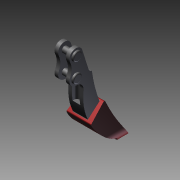
# Autodesk Inventor part: 205-S-HG
Saved by Autodesk Inventor 2011 SP1 (Build 150282100, 282)
## iProperties
Created: 2017-03-01
Part Number: 205-S-HG
Catalog Web Link: www.cadenas.de
Description: HG-SU-Handgriff
Vendor: DESTACO
Document SubType Name: Modeling
Designer: psAdmin
Manufacturer: DESTACO
Mass: 1.83339 g
Surface Area: 15.2284 cm^2
Volume: 1.83339 cm^3
Density: 1 g/cm^3
Category: PARTsolutions
Company: DESTACO
Title: 205-S-HG
Author: Cadenas PARTsolutions
Comments: Handgriff
PSOL_IDENT_0: {$CADENAS_DATA\23d-libs\destaco\destaco_gmbh\man_spann\horizontalspanner\standard\su_parts\handgriff
PSOL_IDENT_1: _su.prj},159 {VTYP=3D},{NB=205-S-HG},{LINA=205-S-HG},{NN=HG-SU},{DATE=20.09.2016 07:53:12},{GEOMDATE=
PSOL_IDENT_2: 01.12.2015 13:32:00},{VERSION=v1},{LINEID=20},{LINESUBID=-1},{WBVAR=}  {NB=205-S-HG},{LINA=205-S-HG}
PSOL_IDENT_3: ,{KT=DUMMY},{MODELL=205-S-HG},{SIZE=1},{MOD=1.000}
NN: HG-SU
NT: Handgriff
NB: 205-S-HG
NBSYN: $MODELL.
LINA: 205-S-HG
MODELL: 205-S-HG
SIZE: 1
MOD: 1.000
SUPPLIER: DESTACO
ARTICLENO: 205-S-HG
BOMINFO: 205-S-HG
CREATOR: CADENAS GmbH
Autodesk Inventor part; units mm, degrees
sketch "Skizze_1" plane through (0, 0, 0) normal (1, 0, 0) x (0, 1, 0)
  arc A0 (2.5764, 8.7074) -> (-2.4358, 6.7351) centre (0, 7.9) ccw
  arc A1 (-2.4358, 1.1649) -> (-2.4358, 6.7351) centre (-8.198, 3.95) ccw
  arc A2 (-2.4358, 1.1649) -> (-0.3542, -2.6767) centre (0, 0) ccw
  line L0 (-0.3542, -2.6767) -> (0.7542, -2.8233)
  arc A3 (3.0986, -5.5855) -> (0.7542, -2.8233) centre (0.4, -5.5) ccw
  line L1 (3.0986, -5.5855) -> (3.0095, -8.3983)
  arc A4 (3.0095, -8.3983) -> (4.8205, -17.1158) centre (22, -9) ccw
  arc A5 (4.7709, -17.3522) -> (4.8205, -17.1158) centre (4.6397, -17.2012) ccw
  line L2 (4.7709, -17.3522) -> (4.4002, -17.6744)
  arc A6 (4.4002, -17.6744) -> (4.2853, -18.2839) centre (4.7282, -18.0518) ccw
  arc A7 (4.2853, -18.2839) -> (14.573, -27.5699) centre (22, -9) ccw
  arc A8 (14.573, -27.5699) -> (17.8933, -31.8025) centre (63, 7) ccw
  line L3 (17.8933, -31.8025) -> (20.1692, -29.8446)
  arc A9 (20.1692, -29.8446) -> (20.2251, -29.1429) centre (19.8432, -29.4656) ccw
  arc A10 (10.72, -13.0698) -> (20.2251, -29.1429) centre (63, 7) ccw
  arc A11 (10.72, -13.0698) -> (9.9251, -12.8717) centre (10.2532, -13.249) ccw
  line L4 (9.9251, -12.8717) -> (9.8793, -12.9115)
  arc A12 (9.5606, -12.8301) -> (9.8793, -12.9115) centre (9.7481, -12.7605) ccw
  arc A13 (6.5211, -0.69) -> (9.5606, -12.8301) centre (63, 7) ccw
  arc A14 (5.1732, 0.4215) -> (6.5211, -0.69) centre (6.7, 0.9) ccw
  line L5 (5.1732, 0.4215) -> (2.5764, 8.7074)
  constraints: 30 point on circle, 15 centre point, 12 end point
extrude "Extrusion1" add sketch "Skizze_1" along normal mid plane 20
sketch "Skizze_2" plane through (0, 0, 0) normal (0, 1, 0) x (-1, 0, 0)
  line L0 (36, 32) -> (-45, 32)
  line L1 (-45, 32) -> (-45, -51)
  line L2 (-45, -51) -> (36, -51)
  line L3 (36, -51) -> (36, 32)
  arc A0 (-5.8716, -24.4048) -> (5.8716, -24.4048) centre (0, -25.16) ccw
  line L4 (5.8716, -24.4048) -> (4.0668, -10.3724)
  line L5 (4.0668, -10.3724) -> (3.075, -10.3724)
  line L6 (3.075, -10.3724) -> (3.075, 10.6)
  line L7 (3.075, 10.6) -> (1.575, 10.6)
  line L8 (1.575, 10.6) -> (1.575, 0.4356)
  arc A1 (-1.575, 0.4356) -> (1.575, 0.4356) centre (0, 0.96) ccw
  line L9 (-1.575, 0.4356) -> (-1.575, 10.6)
  line L10 (-1.575, 10.6) -> (-3.075, 10.6)
  line L11 (-3.075, 10.6) -> (-3.075, -10.3724)
  line L12 (-3.075, -10.3724) -> (-4.0668, -10.3724)
  line L13 (-4.0668, -10.3724) -> (-5.8716, -24.4048)
  constraints: 28 end point, 4 point on circle, 2 centre point
extrude "Extrusion2" cut sketch "Skizze_2" along normal mid plane 100
sketch "Skizze_3" plane through (0, 0, 0) normal (0, 0, 1) x (1, 0, 0)
  line L0 (-32, -32) -> (42, -32)
  line L1 (42, -32) -> (42, 46)
  line L2 (42, 46) -> (-32, 46)
  line L3 (-32, 46) -> (-32, -32)
  line L4 (-3.075, 17.3) -> (-3.075, -2.7)
  line L5 (-3.075, -2.7) -> (-1.575, -2.7)
  line L6 (-1.575, -2.7) -> (-1.575, 4)
  arc A0 (-0.575, 5) -> (-1.575, 4) centre (-0.575, 4) ccw
  line L7 (-0.575, 5) -> (0.575, 5)
  arc A1 (1.575, 4) -> (0.575, 5) centre (0.575, 4) ccw
  line L8 (1.575, 4) -> (1.575, -2.7)
  line L9 (1.575, -2.7) -> (3.075, -2.7)
  line L10 (3.075, -2.7) -> (3.075, 17.3)
  line L11 (3.075, 17.3) -> (-3.075, 17.3)
  constraints: 24 end point, 4 point on circle, 2 centre point
extrude "Extrusion3" cut sketch "Skizze_3" along normal mid plane 24
sketch "Skizze_4" plane through (0, 0, 0) normal (0, -0.7547096, -0.656059) x (1, 0, 0)
  line L0 (-8.075, 33.7744) -> (-8.075, -16.2256)
  line L1 (-8.075, -16.2256) -> (-3.075, -16.2256)
  line L2 (-3.075, -16.2256) -> (-3.075, 30)
  line L3 (-3.075, 30) -> (3.075, 30)
  line L4 (3.075, 30) -> (3.075, -16.2256)
  line L5 (3.075, -16.2256) -> (8.075, -16.2256)
  line L6 (8.075, -16.2256) -> (8.075, 33.7744)
  line L7 (8.075, 33.7744) -> (-8.075, 33.7744)
  constraints: 16 end point
extrude "Extrusion4" cut sketch "Skizze_4" along normal mid plane 20
sketch "Skizze_5" plane through (0, 0, 0) normal (0, 1, 0) x (-1, 0, 0)
  line L0 (3.8624, 0) -> (-3.8624, 0)
  line L1 (-3.8624, 0) -> (-3.8624, 1.405)
  arc A0 (-3.3624, 1.905) -> (-3.8624, 1.405) centre (-3.3624, 1.405) ccw
  line L2 (-3.3624, 1.905) -> (-3.075, 1.905)
  line L3 (-3.075, 1.905) -> (-3.075, 1.6065)
  arc A1 (-3.075, 1.6065) -> (-2.675, 1.2065) centre (-2.675, 1.6065) ccw
  line L4 (-2.675, 1.2065) -> (2.675, 1.2065)
  arc A2 (2.675, 1.2065) -> (3.075, 1.6065) centre (2.675, 1.6065) ccw
  line L5 (3.075, 1.6065) -> (3.075, 1.905)
  line L6 (3.075, 1.905) -> (3.3624, 1.905)
  arc A3 (3.8624, 1.405) -> (3.3624, 1.905) centre (3.3624, 1.405) ccw
  line L7 (3.8624, 1.405) -> (3.8624, 0)
  line L8 (3.8624, 0) -> (-3.8624, 0)
  constraints: 18 end point, 8 point on circle, 4 centre point
sketch "Skizze_6" plane through (0, 0, 0) normal (0, 1, 0) x (-1, 0, 0)
  line L0 (3.8624, 7.9) -> (-3.8624, 7.9)
  line L1 (-3.8624, 7.9) -> (-3.8624, 9.305)
  arc A0 (-3.3624, 9.805) -> (-3.8624, 9.305) centre (-3.3624, 9.305) ccw
  line L2 (-3.3624, 9.805) -> (-3.075, 9.805)
  line L3 (-3.075, 9.805) -> (-3.075, 9.5065)
  arc A1 (-3.075, 9.5065) -> (-2.675, 9.1065) centre (-2.675, 9.5065) ccw
  line L4 (-2.675, 9.1065) -> (2.675, 9.1065)
  arc A2 (2.675, 9.1065) -> (3.075, 9.5065) centre (2.675, 9.5065) ccw
  line L5 (3.075, 9.5065) -> (3.075, 9.805)
  line L6 (3.075, 9.805) -> (3.3624, 9.805)
  arc A3 (3.8624, 9.305) -> (3.3624, 9.805) centre (3.3624, 9.305) ccw
  line L7 (3.8624, 9.305) -> (3.8624, 7.9)
  line L8 (3.8624, 7.9) -> (-3.8624, 7.9)
  constraints: 18 end point, 8 point on circle, 4 centre point
revolve "Revolution1" add sketch "Skizze_5" angle 360 about axis through (-3.8624, 0, 0) along (-1, 0, 0)
revolve "Revolution2" add sketch "Skizze_6" angle 360 about axis through (-3.8624, 0, 7.9) along (-1, 0, 0)
ref_plane "HG1_XY" through (0, 0, 0) normal (1, 0, 0) x (0, 0, -1)
ref_plane "HG1_YZ" through (0, 0, 0) normal (0, 0, -1) x (0, 1, 0)
ref_plane "HG1_ZX" through (0, 0, 0) normal (0, 1, 0) x (1, 0, 0)
ref_plane "HG2_XY" through (0, 0, 7.9) normal (1, 0, 0) x (0, 0, -1)
ref_plane "HG2_YZ" through (0, 0, 7.9) normal (0, 0, -1) x (0, 1, 0)
ref_plane "HG2_ZX" through (0, 0, 7.9) normal (0, 1, 0) x (1, 0, 0)
ref_plane "end_XY" through (0, 18.733, -31.08) normal (1, 0, 0) x (0, 0, -1)
ref_plane "end_YZ" through (0, 18.733, -31.08) normal (0, 0, -1) x (0, 1, 0)
ref_plane "end_ZX" through (0, 18.733, -31.08) normal (0, 1, 0) x (1, 0, 0)
body "Solid1"
